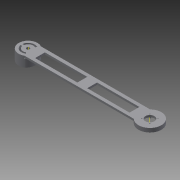
# Autodesk Inventor part: SmallTubeMold
Saved by Autodesk Inventor 2015 (Build 190159000, 159)
## iProperties
Created: 2018-05-03
Part Number: SmallTubeMold
Material: Generic
Document SubType Name: Modeling
Designer: HP USER
Density: 1 g/cm^3
Appearance: Default
Author: HP USER
Autodesk Inventor part; units mm, degrees
ref_plane "YZ Plane" through (0, 0, 0) normal (1, 0, 0) x (0, 1, 0)
ref_plane "XZ Plane" through (0, 0, 0) normal (0, 1, 0) x (-1, 0, 0)
ref_plane "XY Plane" through (0, 0, 0) normal (0, 0, 1) x (1, 0, 0)
sketch "Sketch1" plane through (0, 0, 0) normal (0, 0, 1) x (1, 0, 0)
  line L0 (-6.9363, -17.3613) -> (18.1305, -12.2293) projected
  line L1 (19.1347, -10.9987) -> (18.1305, -12.2293) projected
  line L2 (19.1347, -10.9987) -> (19.1347, 10.9987) projected
  line L3 (18.1305, 12.2293) -> (19.1347, 10.9987) projected
  line L4 (18.1305, 12.2293) -> (-6.9363, 17.3613) projected
  arc A0 (-6.9363, 17.3613) -> (-6.9363, -17.3613) centre (-16.8653, 0) ccw projected
  circle A1 centre (-16.8653, 0) radius 11.5 projected
  arc A2 (6.729, 10.492) -> (9.5926, 10.492) centre (8.1608, 8.692) ccw projected
  line L5 (6.729, 10.492) -> (9.5926, 10.492) projected
  line L6 (9.5932, -10.5127) -> (6.7297, -10.5127) projected
  arc A3 (9.5932, -10.5127) -> (6.7297, -10.5127) centre (8.1614, -8.7127) ccw projected
  line L7 (14.1305, -17.1312) -> (20.3288, -15.8622)
  line L8 (20.3288, -15.8622) -> (23.1347, -12.4236)
  line L9 (23.1347, -12.4236) -> (23.1347, 12.4236)
  line L10 (23.1347, 12.4236) -> (20.3288, 15.8622)
  line L11 (20.3288, 15.8622) -> (14.1305, 17.1312)
  arc A4 (-5.5358, 21.1575) -> (-5.5358, -21.1575) centre (-16.8653, 0) ccw
  line L12 (-5.5358, -21.1575) -> (-5.5358, 21.1575)
  point P0 (0, 0)
  dimension "d0" = 4
  constraints: 12 end point, 2 point on circle, 2 point on line, 1 centre point, 2 other
  measures "d0" radial gap between concentric circles of A0 A4
ref_plane "Work Plane1" through (286.5773, 10.2335, 18) normal (0, 0, 1) x (1, 0, 0)
extrude "Extrusion1" add sketch "Sketch1" along normal up to surface (18 mm away)
sketch "Sketch2" plane through (-16.8653, 0, 18) normal (0, 0, 1) x (1, 0, 0)
  line L0 (303.4426, -24.2629) -> (277, -17.6613) projected
  line L1 (277, 17.6613) -> (303.4426, 24.2629) projected
  line L2 (315.2479, -8.183) -> (314.3455, -8.7476) projected
  arc A0 (321.6657, 8.6432) -> (318.1257, 12.1509) centre (319.753, 10.253) ccw projected
  arc A1 (318.1257, -12.1509) -> (321.6657, -8.6432) centre (319.753, -10.253) ccw projected
  arc A2 (296.9664, -9.2288) -> (301.6459, -9.5496) centre (299.247, -10.253) ccw projected
  arc A3 (301.6459, 9.5496) -> (296.9664, 9.2288) centre (299.247, 10.253) ccw projected
  circle A4 centre (319.753, 10.253) radius 2.5
  circle A5 centre (319.753, -10.253) radius 2.5
  circle A6 centre (299.247, -10.253) radius 2.5
  circle A7 centre (299.247, 10.253) radius 2.5
  line L3 (299.247, -10.253) -> (319.753, 10.253)
  line L4 (319.753, -10.253) -> (299.247, 10.253)
  circle A8 centre (309.5, 0) radius 11.5
  circle A9 centre (309.5, 0) radius 25
  line L5 (277, -17.6613) -> (277, 17.6613)
  line L6 (34.9958, -12.2293) -> (11.3295, -17.0746) projected
  line L7 (36, -10.9987) -> (34.9958, -12.2293) projected
  line L8 (36, 10.9987) -> (36, -10.9987) projected
  line L9 (34.9958, 12.2293) -> (36, 10.9987) projected
  line L10 (11.3295, 17.0746) -> (34.9958, 12.2293) projected
  line L11 (11.3295, 21.1575) -> (11.3295, 17.0746) projected
  arc A10 (11.3295, 21.1575) -> (11.3295, -21.1575) centre (0, 0) ccw projected
  line L12 (11.3295, -17.0746) -> (11.3295, -21.1575) projected
  line L13 (26.4579, 10.492) -> (23.5943, 10.492) projected
  arc A11 (23.5943, 10.492) -> (26.4579, 10.492) centre (25.0261, 8.692) ccw projected
  arc A12 (26.4586, -10.5127) -> (23.595, -10.5127) centre (25.0268, -8.7127) ccw projected
  line L14 (23.595, -10.5127) -> (26.4586, -10.5127) projected
  point P0 (16.8653, 0)
  dimension "d3" = 23
  dimension "d4" = 50
  constraints: 6 end point, 5 coincident, 2 centre point, 1 midpoint, 12 other
  measures "d3" diameter of A8
  measures "d4" diameter of A9
extrude "Extrusion2" add sketch "Sketch2" along normal blind 5
sketch "Sketch3" plane through (0, 0, 0) normal (0, 0, -1) x (-1, 0, 0)
  arc A0 (6.9363, -17.3613) -> (6.9363, 17.3613) centre (16.8653, 0) ccw projected
  arc A1 (5.5358, -21.1575) -> (5.5358, 21.1575) centre (16.8653, 0) ccw projected
  line L0 (5.5358, -17.0746) -> (5.5358, -21.1575) projected
  line L1 (5.5358, 21.1575) -> (5.5358, 17.0746) projected
  line L2 (5.5358, -17.0746) -> (6.9363, -17.3613)
  line L3 (5.5358, 17.0746) -> (6.9363, 17.3613)
  circle A2 centre (16.8653, 0) radius 11.5 projected
  point P0 (0, 0)
  constraints: 4 end point
extrude "Extrusion3" add sketch "Sketch3" along normal blind 3
sketch "Sketch4" plane through (292.6347, 0, 18) normal (0, 0, -1) x (-1, 0, 0)
  circle A0 centre (0, 0) radius 25 projected
  arc A1 (20.3041, 20.7061) -> (20.3041, -20.7061) centre (0, 0) ccw
  line L0 (32.5, 17.6613) -> (6.0574, 24.2629) projected
  line L1 (6.0574, -24.2629) -> (32.5, -17.6613) projected
  line L2 (20.3041, 20.7061) -> (6.0574, 24.2629)
  line L3 (20.3041, -20.7061) -> (6.0574, -24.2629)
  arc A2 (6.0574, 24.2629) -> (6.0574, -24.2629) centre (0, 0) ccw
  point P0 (292.6347, 0)
  dimension "d9" = 4
  constraints: 4 end point, 4 point on circle, 2 centre point, 2 point on line
  measures "d9" radial gap between concentric circles of A0 A1
extrude "Extrusion4" add sketch "Sketch4" along normal blind 5 contours L0 A2 L1 A1
sketch "Sketch5" plane through (292.6347, 0, 23) normal (0, 0, 1) x (1, 0, 0)
  line L0 (-6.0574, 24.2629) -> (-20.3041, 20.7061) projected
  arc A0 (-6.0574, -24.2629) -> (-6.0574, 24.2629) centre (0, 0) ccw projected
  line L1 (-20.3041, -20.7061) -> (-6.0574, -24.2629) projected
  arc A1 (-20.3041, -20.7061) -> (-20.3041, 20.7061) centre (0, 0) ccw projected
  line L2 (-20.3041, 20.7061) -> (-20.3041, -20.7061)
  circle A2 centre (0, 0) radius 11.5 projected
  circle A3 centre (-10.253, 10.253) radius 2.5 projected
  circle A4 centre (-10.253, -10.253) radius 2.5 projected
  circle A5 centre (10.253, -10.253) radius 2.5 projected
  circle A6 centre (10.253, 10.253) radius 2.5 projected
  circle A7 centre (0, 0) radius 25 projected
  point P0 (-292.6347, 0)
  constraints: 2 end point
extrude "Extrusion5" add sketch "Sketch5" against normal up to surface (5 mm away) contours A0 L1 L2 A7 L0 | L0 A1 L1 A0 | A7 L2 picked at (-17.3694, 0)
sketch "Sketch6" plane through (272.3305, -20.7061, 23) normal (-1, 0, 0) x (0, 0, 1)
  line L0 (0, 35.2918) -> (-5, 35.2918) projected
  line L1 (0, 41.4122) -> (0, 35.2918) projected
  line L2 (0, 41.4122) -> (-5, 41.4122) projected
  line L3 (-5, 35.2918) -> (-5, 41.4122) projected
  line L4 (-5, 6.1204) -> (0, 6.1204) projected
  line L5 (-5, 0) -> (-5, 6.1204) projected
  line L6 (0, 0) -> (-5, 0) projected
  line L7 (0, 6.1204) -> (0, 0) projected
  line L8 (0, 41.4122) -> (-5, 41.4122)
  line L9 (-5, 41.4122) -> (-5, 0)
  line L10 (-5, 0) -> (0, 0)
  line L11 (0, 0) -> (0, 41.4122)
  point P0 (-23, 20.7061)
  constraints: 8 end point
extrude "Extrusion6" add sketch "Sketch6" along normal up to surface (277.8663 mm away)
sketch "Sketch7" plane through (-16.8653, 0, 18) normal (0, 0, -1) x (-1, 0, 0)
  circle A0 centre (-299.247, -10.253) radius 2.5 projected
  circle A1 centre (-319.753, -10.253) radius 2.5 projected
  circle A2 centre (-319.753, -10.253) radius 2.5 projected
  circle A3 centre (-299.247, 10.253) radius 2.5 projected
  circle A4 centre (-319.753, 10.253) radius 2.5 projected
  point P0 (-16.8653, 0)
extrude "Extrusion7" add sketch "Sketch7" along normal blind 3 and the other way blind 5
sketch "Sketch8" plane through (0, 0, 0) normal (0, 0, -1) x (-1, 0, 0)
  line L0 (5.5358, 21.1575) -> (-20.2672, 21.1575)
  line L1 (-20.2672, 21.1575) -> (-20.2672, -21.1575)
  line L2 (-20.2672, -21.1575) -> (5.5358, -21.1575)
  line L3 (5.5358, -21.1575) -> (5.5358, 21.1575)
  point P0 (0, 0)
  point P1 (5.5358, -17.0746)
  point P2 (5.5358, 17.0746)
  point P3 (5.5358, -21.1575)
  constraints: 8 end point
extrude "Extrusion8" cut sketch "Sketch8" against normal up to surface (18 mm away)
sketch "Sketch9" plane through (-16.8653, 0, -3) normal (0, 0, -1) x (-1, 0, 0)
  circle A0 centre (0, 0) radius 11.5 projected
  circle A1 centre (0, 0) radius 4
  point P0 (-16.8653, 0)
  dimension "d24" = 8
  constraints: 1 centre point, 1 coincident
  measures "d24" diameter of A1
extrude "Extrusion9" cut sketch "Sketch9" against normal blind 40.75 contours A1
sketch "Sketch10" plane through (-16.8653, 0, -3) normal (0, 0, -1) x (-1, 0, 0)
  circle A0 centre (0, 0) radius 4 projected
  circle A1 centre (0, 0) radius 8.5
  circle A2 centre (0, 0) radius 11.5 projected
  point P0 (-16.8653, 0)
  dimension "d27" = 17
  constraints: 1 centre point, 1 coincident
  measures "d27" diameter of A1
extrude "Extrusion10" cut sketch "Sketch10" against normal up to surface (3 mm away) contours A2
sketch "Sketch11" plane through (0, 0, 0) normal (0, 0, -1) x (-1, 0, 0)
  arc A0 (6.9363, -17.3613) -> (6.9363, 17.3613) centre (16.8653, 0) ccw projected
  line L0 (10.4115, -11.2849) -> (8.4257, -14.7571)
  line L1 (10.4115, 11.2849) -> (8.4257, 14.7571)
  line L2 (33.7004, -2.3626) -> (29.6488, -2.3626)
  line L3 (29.6488, 2.3626) -> (33.7004, 2.3626)
  arc A1 (8.4257, -14.7571) -> (33.7004, -2.3626) centre (16.8653, 0) ccw
  arc A2 (33.7004, 2.3626) -> (8.4257, 14.7571) centre (16.8653, 0) ccw
  arc A3 (10.4115, -11.2849) -> (29.6488, -2.3626) centre (16.8653, 0) ccw
  arc A4 (29.6488, 2.3626) -> (10.4115, 11.2849) centre (16.8653, 0) ccw
  point P0 (0, 0)
  point P1 (31.8653, 0)
  constraints: 8 end point, 8 point on circle, 4 centre point
extrude "Extrusion11" cut sketch "Sketch11" against normal blind 40.75
sketch "Sketch12" plane through (-16.8653, 0, 18) normal (0, 0, -1) x (-1, 0, 0)
  line L0 (-289.1959, 20.7061) -> (-11.3295, 20.7061) projected
  line L1 (-289.1959, -20.7061) -> (-11.3295, -20.7061) projected
  line L2 (-289.1959, 20.7061) -> (-11.3295, 20.7061) projected
  line L3 (-150.2627, 20.7061) -> (-150.2627, -20.7061)
  line L4 (-30.2627, 12.5) -> (-30.2627, -12.5)
  line L5 (-270.2627, -12.5) -> (-270.2627, 12.5)
  line L6 (-137.7627, 12.5) -> (-137.7627, -12.5)
  line L7 (-162.7627, -12.5) -> (-162.7627, 12.5)
  line L8 (-270.2627, 12.5) -> (-162.7627, 12.5)
  line L9 (-137.7627, 12.5) -> (-30.2627, 12.5)
  line L10 (-30.2627, -12.5) -> (-137.7627, -12.5)
  line L11 (-162.7627, -12.5) -> (-270.2627, -12.5)
  point P0 (-16.8653, 0)
  point P1 (-150.2627, 0)
  point P2 (-150.2627, 0)
  dimension "d35" = 25
  constraints: 18 end point, 3 midpoint
  measures "d35" distance of L4.start L4.end
extrude "Extrusion12" cut sketch "Sketch12" against normal up to surface (5 mm away)
sketch "Sketch13" plane through (-16.8653, 0, 18) normal (0, 0, -1) x (-1, 0, 0)
  line L0 (-155.1522, 3) -> (-145.1522, 3)
  line L1 (-145.1522, -3) -> (-155.1522, -3)
  line L2 (-155.1522, -3) -> (-155.1522, 3)
  line L3 (-145.1522, 3) -> (-145.1522, 20.7061)
  line L4 (-145.1522, -3) -> (-145.1522, -20.7061)
  line L5 (-289.1959, 20.7061) -> (-11.3295, 20.7061) projected
  line L6 (-289.1959, -20.7061) -> (-11.3295, -20.7061) projected
  line L7 (-145.1522, 20.7061) -> (-145.1522, 87.1376)
  line L8 (-145.1522, 87.1376) -> (54.4228, 87.1376)
  line L9 (54.4228, 87.1376) -> (54.4228, -46.013)
  line L10 (54.4228, -46.013) -> (-145.1522, -46.013)
  line L11 (-145.1522, -46.013) -> (-145.1522, -20.7061)
  line L12 (-145.1522, 87.1376) -> (-367.5334, 87.1376)
  line L13 (-145.1522, 87.1376) -> (77.2289, 87.1376) construction
  line L14 (-367.5334, 87.1376) -> (-367.5334, -46.013)
  line L15 (-367.5334, -46.013) -> (-145.1522, -46.013)
  point P0 (-16.8653, 0)
  point P1 (-162.7627, 12.5)
  point P2 (-150.1522, 0)
  dimension "d42" = 90
  dimension "d43" = 90
  dimension "d44" = 90
  dimension "d45" = 180
  constraints: 28 end point, 4 point on line, 1 collinear, 1 horizontal
  measures "d42" angle of L7 L8
  measures "d43" angle of L8 L9
  measures "d44" angle of L9 L10
  measures "d45" angle of L12 L13
extrude "StlSplit" [suppressed]
sketch "Sketch14" plane through (282.3816, 10.253, 15) normal (0, 0, -1) x (-1, 0, 0)
  circle A0 centre (0, 0) radius 2.5 projected
  circle A1 centre (-20.5061, 0) radius 2.5 projected
  circle A2 centre (-20.5061, -20.5061) radius 2.5 projected
  circle A3 centre (0, -20.5061) radius 2.5 projected
  circle A4 centre (-20.5061, 0) radius 2.5 projected
  circle A5 centre (-20.5061, 0) radius 1
  circle A6 centre (0, 0) radius 2.5 projected
  circle A7 centre (0, 0) radius 1
  circle A8 centre (-20.5061, -20.5061) radius 2.5 projected
  circle A9 centre (-20.5061, -20.5061) radius 1
  circle A10 centre (0, -20.5061) radius 2.5 projected
  circle A11 centre (0, -20.5061) radius 1
  point P0 (282.3816, -10.253)
  dimension "d51" = 2
  dimension "d52" = 2
  dimension "d53" = 2
  dimension "d54" = 2
  constraints: 4 centre point, 4 coincident
  measures "d51" diameter of A5
  measures "d52" diameter of A7
  measures "d53" diameter of A9
  measures "d54" diameter of A11
extrude "Extrusion14" cut sketch "Sketch14" against normal blind 40.75 contours A5 | A7 | A9 | A11
sketch "Sketch15" plane through (0, 0, 0) normal (0, 0, -1) x (-1, 0, 0)
  arc A0 (8.4257, -14.7571) -> (33.7004, -2.3626) centre (16.8653, 0) ccw projected
  line L0 (8.4257, -14.7571) -> (10.4115, -11.2849) projected
  arc A1 (10.4115, -11.2849) -> (29.6488, -2.3626) centre (16.8653, 0) ccw projected
  line L1 (29.6488, -2.3626) -> (33.7004, -2.3626) projected
  arc A2 (29.6488, 2.3626) -> (10.4115, 11.2849) centre (16.8653, 0) ccw projected
  line L2 (10.4115, 11.2849) -> (8.4257, 14.7571) projected
  arc A3 (33.7004, 2.3626) -> (8.4257, 14.7571) centre (16.8653, 0) ccw projected
  line L3 (33.7004, 2.3626) -> (29.6488, 2.3626) projected
  circle A4 centre (16.8653, 0) radius 8.5 projected
  line L4 (5.5358, -17.0746) -> (5.5358, 17.0746) projected
  line L5 (5.5358, -17.0746) -> (6.9363, -17.3613) projected
  arc A5 (6.9363, -17.3613) -> (6.9363, 17.3613) centre (16.8653, 0) ccw projected
  line L6 (6.9363, 17.3613) -> (5.5358, 17.0746) projected
  point P0 (0, 0)
extrude "Extrusion15" cut sketch "Sketch15" against normal blind 17
sketch "Sketch16" plane through (0, 0, -3) normal (0, 0, -1) x (-1, 0, 0)
  circle A0 centre (16.8653, 0) radius 6
  arc A1 (16.8653, 20) -> (16.8653, -20) centre (25.7499, 0) ccw
  arc A2 (16.8653, -20) -> (16.8653, 20) centre (16.8653, 0) ccw
  circle A3 centre (16.8653, 0) radius 4 projected
  arc A4 (4.0089, -20.2661) -> (4.0089, 20.2661) centre (16.8653, 0) ccw
  arc A5 (4.0089, 20.2661) -> (4.0089, -20.2661) centre (25.7499, 0) ccw
  point P0 (0, 0)
  constraints: 8 point on circle, 5 centre point
extrude "Extrusion16" add sketch "Sketch16" against normal up to surface (20 mm away) contours A5 A4
sketch "Sketch17" plane through (-16.8653, 0, -3) normal (0, 0, -1) x (-1, 0, 0)
  circle A0 centre (0, 0) radius 8.5 projected
  circle A1 centre (0, 0) radius 4 projected
  point P0 (-16.8653, 0)
extrude "Extrusion17" cut sketch "Sketch17" against normal up to surface (20 mm away)
body "Solid1"
